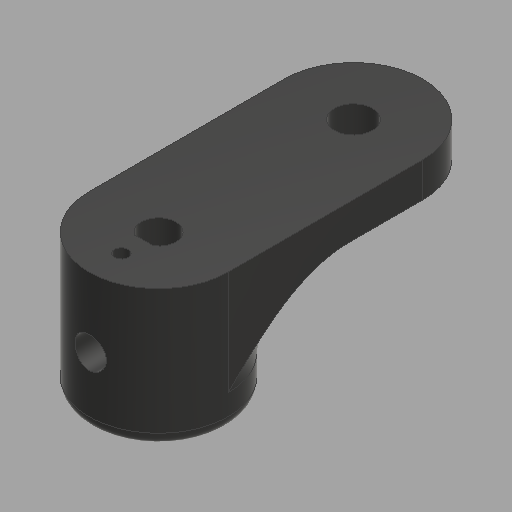
# Autodesk Inventor part: BT001_trajan20_21
Saved by Autodesk Inventor 2023 (Build 270158000, 158)
## iProperties
Company: HTBLA Kaindorf
RuleStatus: InUse
Created: 2022-08-07
Part Number: BT001_trajan20_21
Project: Zeichenmaschine_v2
Material: Kunststoff, undurchsichtig Schwarz
Description: gelenk 1
Document SubType Name: Modeling
Designer: trajan20
Density: 0.952 g/cm^3
Appearance: Glatt - Schwarz
Mass: 8.30497 g
Surface Area: 38.2792 cm^2
Volume: 8.72371 cm^3
AfterDocNew0: iProperties-Editor_aufrufen
Author: jan
Keywords: 2021
Autodesk Inventor part; units mm, degrees
ref_plane "YZ Plane" through (0, 0, 0) normal (1, 0, 0) x (0, 1, 0)
ref_plane "XZ Plane" through (0, 0, 0) normal (0, 1, 0) x (-1, 0, 0)
ref_plane "XY Plane" through (0, 0, 0) normal (0, 0, 1) x (1, 0, 0)
sketch "Skizze3" plane through (0, 0, 0) normal (0, 0, 1) x (1, 0, 0)
  line L0 (0, 0) -> (-28, 0) construction
  line L1 (0, 10) -> (-28, 10)
  line L2 (-28, -10) -> (0, -10)
  arc A0 (0, -10) -> (0, 10) centre (0, 0) ccw
  arc A1 (-28, 10) -> (-28, -10) centre (-28, 0) ccw
  circle A2 centre (0, 0) radius 2.5
  circle A3 centre (-28, 0) radius 2.75
  point P0 (-14, 0)
  point P1 (-40, 0)
  dimension "d4" = 28
  dimension "d5" = 20
  dimension "d6" = 5.5
  dimension "d7" = 5
  dimension "d8" = 40
  constraints: 8 end point, 4 centre point, 4 point on circle, 4 tangent, 2 coincident, 1 horizontal, 1 midpoint, 1 parallel, 1 point on line
  measures "d4" distance of L0.end L0.start
  measures "d5" distance between parallel lines of L2 L1
  measures "d6" diameter of A3
  measures "d7" diameter of A2
  measures "d8" distance of L0.start point (-40, 0)
extrude "Extrusion3" add sketch "Skizze3" along normal blind 5
sketch "Skizze5" plane through (0, 0, 0) normal (0, 0, -1) x (-1, 0, 0)
  circle A0 centre (0, 0) radius 2.5 projected
  circle A1 centre (0, 0) radius 10
  line L0 (0, 10) -> (28, 10) projected
  constraints: 1 coincident, 1 horizontal, 1 vertical alignment, 1 other
extrude "Extrusion4" add sketch "Skizze5" along normal blind 15
fillet "Rundung1" radius 10 2 edges at (-7.0711, 7.0711, 0) (-7.0711, -7.0711, 0)
ref_plane "Arbeitsebene1" through (10, 0, 5) normal (1, 0, 0) x (0, 1, 0)
sketch "Skizze7" plane through (10, 0, 5) normal (1, 0, 0) x (0, 1, 0)
  line L0 (-2.5, 0) -> (-2.5, -20) projected
  line L1 (-2.5, 0) -> (-2.5, -20) projected
  line L2 (2.5, 0) -> (2.5, -20) projected
  line L3 (2.5, 0) -> (2.5, -20) projected
  line L4 (0, -6.4797) -> (0, -2.8398) construction
  line L5 (-10, -20) -> (10, -20) projected
  line L6 (-10, -5) -> (10, -5) projected
  point P0 (0, -5)
  point P1 (0, -10)
  point P2 (0, -15)
  dimension "d30" = 5
  dimension "d31" = 5
  constraints: 3 point on line, 2 end point, 1 vertical
  measures "d30" distance from line of L5 point (0, -15)
  measures "d31" distance from line of L6 point (0, -10)
hole "Bohrung3" at (10, 0, -5) direction (-1, 0, 0) diameter 4.5 end up to face face through (0, 0, 0) facing (0, 0, 1) round with radius 2.5 far side no
fillet "Rundung2" radius 2 1 edges at (10, 0, -15)
sketch "Skizze8" plane through (0, 0, -15) normal (0, 0, -1) x (-1, 0, 0)
  line L0 (-4.2, -3.565) -> (-6.5, -3.565)
  line L1 (-6.5, -3.565) -> (-6.5, 3.565)
  line L2 (-6.5, 3.565) -> (-4.2, 3.565)
  line L3 (-4.2, 3.565) -> (-4.2, -3.565)
  point P0 (0, 0)
  point P1 (-6.5, 0)
  dimension "d40" = 7.13
  dimension "d41" = 2.3
  dimension "d42" = 4.2
  constraints: 8 end point, 2 parallel, 1 horizontal, 1 horizontal alignment, 1 midpoint, 1 perpendicular
  measures "d40" distance between parallel lines of L0 L2
  measures "d41" distance between parallel lines of L3 L1
  measures "d42" distance from line of point (0, 0) L3
extrude "Extrusion5" cut sketch "Skizze8" against normal blind 13.7
sketch "Skizze9" plane through (0, 0, 5) normal (0, 0, 1) x (1, 0, 0)
  circle A0 centre (0, 0) radius 2.5 projected
  line L0 (2.1, 1.3565) -> (2.1, -1.3565)
  line L1 (4.2, 3.565) -> (4.2, -3.565) projected
  line L2 (6.5, -3.565) -> (6.5, 3.565) projected
  line L3 (6.5, 3.565) -> (4.2, 3.565) projected
  line L4 (4.2, -3.565) -> (6.5, -3.565) projected
  circle A1 centre (5.35, 0) radius 1
  point P0 (4.2, 0)
  point P1 (5.35, -3.565)
  dimension "d45" = 2.1
  dimension "d48" = 2
  constraints: 2 end point, 2 midpoint, 2 point on circle, 1 centre point, 1 coincident, 1 horizontal alignment, 1 vertical, 1 vertical alignment
  measures "d45" distance from line of point (0, 0) L0
  measures "d48" diameter of A1
extrude "Extrusion6" add sketch "Skizze9" against normal blind 15 contours A0 L0 picked at (2.1732, -0.3109)
extrude "Extrusion7" cut sketch "Skizze9" against normal blind 15 contours A1
equation "\"d31\" = d30"
